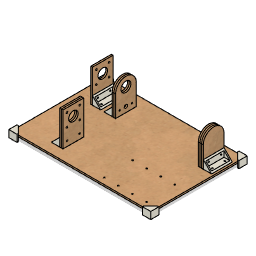
Frame (Autodesk Fusion 360 design; units mm, degrees)
Autodesk Fusion 360 part; units mm, degrees
note: some values were not read from the file. Chosen so that the rebuilt part matches the saved one: a direction; where a step ends. Set by a fixed rule: which sketch regions a step uses.
(part 1 of 2)
sketch "Sketch1" plane through (0, 0, 0) normal (0, 1, 0) x (1, 0, 0)
  line L0 (-148.1327, 87.8458) -> (188.6673, 87.8458)
  line L1 (188.6673, 87.8458) -> (188.6673, -139.1542)
  line L2 (188.6673, -139.1542) -> (-148.1327, -139.1542)
  line L3 (-148.1327, -139.1542) -> (-148.1327, 87.8458)
  line L4 (400.9033, 37.8458) -> (350, 37.8458) construction
  line L5 (350, 37.8458) -> (-250, 37.8458) construction
  line L6 (400, -89.1542) -> (-263.6567, -89.1542) construction
  line L7 (151.7073, 62.8058) -> (163.6273, 62.8058)
  line L8 (163.6273, 62.8058) -> (163.6273, 12.8858)
  line L9 (163.6273, 12.8858) -> (151.7073, 12.8858)
  line L10 (151.7073, 12.8858) -> (151.7073, 62.8058)
  line L11 (-56.2127, 62.8058) -> (-48.2927, 62.8058)
  line L12 (-48.2927, 62.8058) -> (-48.2927, 12.8858)
  line L13 (-48.2927, 12.8858) -> (-56.2127, 12.8858)
  line L14 (-56.2127, 12.8858) -> (-56.2127, 62.8058)
  line L15 (-108.1327, 62.8058) -> (-104.2127, 62.8058)
  line L16 (-104.2127, 62.8058) -> (-104.2127, 12.8858)
  line L17 (-104.2127, 12.8858) -> (-108.1327, 12.8858)
  line L18 (-108.1327, 12.8858) -> (-108.1327, 62.8058)
  line L19 (-56.2127, -64.1942) -> (-48.2927, -64.1942)
  line L20 (-48.2927, -64.1942) -> (-48.2927, -114.1142)
  line L21 (-48.2927, -114.1142) -> (-56.2127, -114.1142)
  line L22 (-56.2127, -114.1142) -> (-56.2127, -64.1942)
  line L23 (155.7073, -64.1942) -> (163.6273, -64.1942)
  line L24 (163.6273, -64.1942) -> (163.6273, -114.1142)
  line L25 (163.6273, -114.1142) -> (155.7073, -114.1142)
  line L26 (155.7073, -114.1142) -> (155.7073, -64.1942)
  line L27 (-108.1327, 46.2192) -> (-104.2127, 46.2192)
  line L28 (-104.2127, 46.2192) -> (-104.2127, 29.4725)
  line L29 (-104.2127, 29.4725) -> (-108.1327, 29.4725)
  line L30 (-108.1327, 29.4725) -> (-108.1327, 46.2192)
  line L31 (-56.2127, 46.2192) -> (-48.2927, 46.2192)
  line L32 (-48.2927, 46.2192) -> (-48.2927, 29.4725)
  line L33 (-48.2927, 29.4725) -> (-56.2127, 29.4725)
  line L34 (-56.2127, 29.4725) -> (-56.2127, 46.2192)
  line L35 (151.7073, 46.2192) -> (163.6273, 46.2192)
  line L36 (163.6273, 46.2192) -> (163.6273, 29.4725)
  line L37 (163.6273, 29.4725) -> (151.7073, 29.4725)
  line L38 (151.7073, 29.4725) -> (151.7073, 46.2192)
  line L39 (-56.2127, -80.7808) -> (-48.2927, -80.7808)
  line L40 (-48.2927, -80.7808) -> (-48.2927, -97.5275)
  line L41 (-48.2927, -97.5275) -> (-56.2127, -97.5275)
  line L42 (-56.2127, -97.5275) -> (-56.2127, -80.7808)
  line L43 (155.7073, -80.7808) -> (163.6273, -80.7808)
  line L44 (163.6273, -80.7808) -> (163.6273, -97.5275)
  line L45 (163.6273, -97.5275) -> (155.7073, -97.5275)
  line L46 (155.7073, -97.5275) -> (155.7073, -80.7808)
  dimension "d4" = 127
  dimension "d5" = 50
  dimension "d6" = 50
  dimension "d7" = 7.92
  dimension "d8" = 11.92
  dimension "d9" = 7.92
  dimension "d10" = 7.92
  dimension "d12" = 49.92
  dimension "d13" = 49.92
  dimension "d14" = 49.92
  dimension "d15" = 49.92
  dimension "d16" = 49.92
  dimension "d17" = 3.92
  dimension "d18" = 24.96
  dimension "d19" = 24.96
  dimension "d20" = 24.96
  dimension "d21" = 24.96
  dimension "d22" = 24.96
  dimension "d23" = 25.04
  dimension "d24" = 7.92
  dimension "d25" = 200
  dimension "d26" = 25.04
  dimension "d27" = 40
  dimension "d28" = 48
  dimension "d455" = 16.7467
  dimension "d456" = 16.5867
  dimension "d457" = 16.7467
  dimension "d458" = 16.5867
  dimension "d459" = 16.7467
  dimension "d460" = 16.5867
  dimension "d461" = 16.5867
  dimension "d462" = 16.7467
  dimension "d463" = 16.5867
  dimension "d464" = 16.7467
  constraint horizontal L0
  constraint vertical L1
  constraint horizontal L2
  constraint vertical L3
  constraint perpendicular L1 L4
  constraint perpendicular L1 L5
  constraint perpendicular L3 L6
  constraint horizontal L7
  constraint vertical L8
  constraint horizontal L9
  constraint vertical L10
  constraint horizontal L11
  constraint vertical L12
  constraint horizontal L13
  constraint vertical L14
  constraint horizontal L15
  constraint vertical L16
  constraint horizontal L17
  constraint vertical L18
  constraint horizontal L19
  constraint vertical L20
  constraint horizontal L21
  constraint vertical L22
  constraint horizontal L23
  constraint vertical L24
  constraint horizontal L25
  constraint vertical L26
  constraint horizontal L27
  constraint vertical L28
  constraint horizontal L29
  constraint vertical L30
  constraint coincident L16 L28.end
  constraint coincident L18 L27.start
  constraint horizontal L31
  constraint vertical L32
  constraint horizontal L33
  constraint vertical L34
  constraint coincident L12 L32.end
  constraint coincident L14 L31.start
  constraint horizontal L35
  constraint vertical L36
  constraint horizontal L37
  constraint vertical L38
  constraint coincident L8 L36.end
  constraint coincident L10 L35.start
  constraint horizontal L39
  constraint vertical L40
  constraint horizontal L41
  constraint vertical L42
  constraint coincident L20 L40.end
  constraint coincident L22 L39.start
  constraint horizontal L43
  constraint vertical L44
  constraint horizontal L45
  constraint vertical L46
  constraint coincident L24 L44.end
  constraint coincident L26 L43.start
  measures "d4" distance of L5 L6
  measures "d5" distance of L2 L6
  measures "d6" distance of L0 L4.end
  measures "d7" distance of L23.start L23.end
  measures "d8" distance of L7.start L7.end
  measures "d9" distance of L11.start L11.end
  measures "d10" distance of L19.start L19.end
  measures "d12" distance of L7.end L8.end
  measures "d13" distance of L23.end L24.end
  measures "d14" distance of L19.end L20.end
  measures "d15" distance of L11.end L12.end
  measures "d16" distance of L15.end L16.end
  measures "d17" distance of L15.start L15.end
  measures "d18" distance of L5 L15.end
  measures "d19" distance of L5 L11.end
  measures "d20" distance of L5 L7.end
  measures "d21" distance of L6 L19.end
  measures "d22" distance of L6 L23.end
  measures "d23" distance of L1 L24
  measures "d24" horizontal distance of L13.end L19.end
  measures "d25" distance of L10 L12
  measures "d26" distance of L1 L8
  measures "d27" distance of L3 L18
  measures "d28" distance of L14 L16
  measures "d455" distance of L27 L29
  measures "d456" distance of L15 L27
  measures "d457" distance of L27 L33
  measures "d458" distance of L11 L31
  measures "d459" distance of L35 L37
  measures "d460" distance of L7.start L35
  measures "d461" distance of L19 L39
  measures "d462" distance of L39 L41
  measures "d463" distance of L23 L43
  measures "d464" distance of L43 L45
extrude "Extrude1" add sketch "Sketch1" along normal blind 4 contours L0 L1 L2 L3 | L8 L10 L35 L36 L37 L38 | L12 L14 L31 L32 L33 L34 | L16 L18 L27 L28 L29 L30 | L20 L22 L39 L40 L41 L42 | L23 L24 L26 L43 | L24 L26 L43 L44 L45 L46 | L24 L25 L26 L45 makes body 1
sketch "Sketch2" plane through (0, 4, 0) normal (0, 1, 0) x (-1, 0, 0)
  line L0 (-163.6273, -12.8858) -> (-151.7073, -12.8858)
  line L1 (-151.7073, -46.2192) -> (-151.7073, -62.8058)
  line L2 (-151.7073, -62.8058) -> (-163.6273, -62.8058)
  line L3 (-163.6273, -62.8058) -> (-163.6273, -46.2192)
  line L4 (48.2927, -12.8858) -> (56.2127, -12.8858)
  line L5 (56.2127, -12.8858) -> (56.2127, -29.4725)
  line L6 (56.2127, -62.8058) -> (48.2927, -62.8058)
  line L7 (48.2927, -29.4725) -> (48.2927, -12.8858)
  line L8 (104.2127, -12.8858) -> (108.1327, -12.8858)
  line L9 (108.1327, -46.2192) -> (108.1327, -62.8058)
  line L10 (108.1327, -62.8058) -> (104.2127, -62.8058)
  line L11 (104.2127, -62.8058) -> (104.2127, -46.2192)
  line L12 (48.2927, 114.1142) -> (56.2127, 114.1142)
  line L13 (56.2127, 114.1142) -> (56.2127, 97.5275)
  line L14 (56.2127, 64.1942) -> (48.2927, 64.1942)
  line L15 (48.2927, 97.5275) -> (48.2927, 114.1142)
  line L16 (148.1327, 139.1542) -> (-188.6673, 139.1542)
  line L17 (-188.6673, 139.1542) -> (-188.6673, -87.8458)
  line L18 (-188.6673, -87.8458) -> (148.1327, -87.8458)
  line L19 (148.1327, -87.8458) -> (148.1327, 139.1542)
  line L20 (-243.4982, -14.4378) -> (-263.4982, -14.4378)
  line L21 (-263.4982, -14.4378) -> (-263.4982, 5.5622)
  line L22 (-263.4982, 5.5622) -> (-243.4982, 5.5622)
  line L23 (-243.4982, 5.5622) -> (-243.4982, -14.4378)
  line L24 (104.2127, -46.2192) -> (108.1327, -46.2192)
  line L25 (104.2127, -29.4725) -> (104.2127, -12.8858)
  line L26 (108.1327, -12.8858) -> (108.1327, -29.4725)
  line L27 (108.1327, -29.4725) -> (104.2127, -29.4725)
  line L28 (56.2127, -29.4725) -> (48.2927, -29.4725)
  line L29 (56.2127, -46.2192) -> (56.2127, -62.8058)
  line L30 (48.2927, -62.8058) -> (48.2927, -46.2192)
  line L31 (48.2927, -46.2192) -> (56.2127, -46.2192)
  line L32 (-163.6273, -46.2192) -> (-151.7073, -46.2192)
  line L33 (-163.6273, -29.4725) -> (-163.6273, -12.8858)
  line L34 (-151.7073, -12.8858) -> (-151.7073, -29.4725)
  line L35 (-151.7073, -29.4725) -> (-163.6273, -29.4725)
  line L36 (56.2127, 97.5275) -> (48.2927, 97.5275)
  line L37 (56.2127, 80.7808) -> (56.2127, 64.1942)
  line L38 (48.2927, 64.1942) -> (48.2927, 80.7808)
  line L39 (48.2927, 80.7808) -> (56.2127, 80.7808)
  dimension "d32" = 20
  dimension "d33" = 20
  constraint horizontal L20
  constraint vertical L21
  constraint horizontal L22
  constraint vertical L23
  measures "d32" distance of L20.start L20.end
  measures "d33" distance of L20.start L22.end
extrude "Extrude2" add sketch "Sketch2" along normal blind 17 separate body contours L20 L21 L22 L23 makes body 2
chamfer "Chamfer1" distance 17 angle 45 1 edges at (263.4982, 12.5, 5.5622) on bodies 2
sketch "Sketch3" plane through (0, 21, 0) normal (0, 1, 0) x (-1, 0, 0)
  line L0 (-246.4982, 5.5622) -> (-263.4982, -11.4378)
  line L1 (-263.4982, -11.4378) -> (-263.4982, -14.4378)
  line L2 (-263.4982, -14.4378) -> (-243.4982, -14.4378)
  line L3 (-243.4982, -14.4378) -> (-243.4982, 5.5622)
  line L4 (-243.4982, 5.5622) -> (-246.4982, 5.5622)
  line L5 (-246.4982, -11.4378) -> (-266.4982, -11.4378)
  line L6 (-266.4982, -11.4378) -> (-266.4982, 8.5622)
  line L7 (-266.4982, 8.5622) -> (-246.4982, 8.5622)
  line L8 (-246.4982, 8.5622) -> (-246.4982, -11.4378)
  dimension "d37" = 3
  dimension "d38" = 3
  dimension "d39" = 20
  dimension "d40" = 20
  constraint horizontal L5
  constraint vertical L6
  constraint horizontal L7
  constraint vertical L8
  measures "d37" distance of L2 L5
  measures "d38" distance of L3 L8
  measures "d39" distance of L6.end L7.end
  measures "d40" distance of L5.end L6.end
extrude "Extrude3" cut sketch "Sketch3" against normal blind 4 from surface at -3 contours L0 L5 L8 | L0 L5 L6 L7 L8 bodies 2
sketch "Sketch4" plane through (0, 4, 0) normal (0, 1, 0) x (-1, 0, 0)
  line L0 (-163.6273, -12.8858) -> (-151.7073, -12.8858)
  line L1 (-151.7073, -46.2192) -> (-151.7073, -62.8058)
  line L2 (-151.7073, -62.8058) -> (-163.6273, -62.8058)
  line L3 (-163.6273, -62.8058) -> (-163.6273, -46.2192)
  line L4 (48.2927, -12.8858) -> (56.2127, -12.8858)
  line L5 (56.2127, -12.8858) -> (56.2127, -29.4725)
  line L6 (56.2127, -62.8058) -> (48.2927, -62.8058)
  line L7 (48.2927, -29.4725) -> (48.2927, -12.8858)
  line L8 (104.2127, -12.8858) -> (108.1327, -12.8858)
  line L9 (108.1327, -46.2192) -> (108.1327, -62.8058)
  line L10 (108.1327, -62.8058) -> (104.2127, -62.8058)
  line L11 (104.2127, -62.8058) -> (104.2127, -46.2192)
  line L12 (48.2927, 114.1142) -> (56.2127, 114.1142)
  line L13 (56.2127, 114.1142) -> (56.2127, 97.5275)
  line L14 (56.2127, 64.1942) -> (48.2927, 64.1942)
  line L15 (48.2927, 97.5275) -> (48.2927, 114.1142)
  line L16 (148.1327, 139.1542) -> (-188.6673, 139.1542)
  line L17 (-188.6673, 139.1542) -> (-188.6673, -87.8458)
  line L18 (-188.6673, -87.8458) -> (148.1327, -87.8458)
  line L19 (148.1327, -87.8458) -> (148.1327, 139.1542)
  line L20 (-250, 50) -> (-270, 50)
  line L21 (-270, 50) -> (-270, 70)
  line L22 (-270, 70) -> (-250, 70)
  line L23 (-250, 70) -> (-250, 50)
  line L24 (104.2127, -46.2192) -> (108.1327, -46.2192)
  line L25 (104.2127, -29.4725) -> (104.2127, -12.8858)
  line L26 (108.1327, -12.8858) -> (108.1327, -29.4725)
  line L27 (108.1327, -29.4725) -> (104.2127, -29.4725)
  line L28 (56.2127, -29.4725) -> (48.2927, -29.4725)
  line L29 (56.2127, -46.2192) -> (56.2127, -62.8058)
  line L30 (48.2927, -62.8058) -> (48.2927, -46.2192)
  line L31 (48.2927, -46.2192) -> (56.2127, -46.2192)
  line L32 (-163.6273, -46.2192) -> (-151.7073, -46.2192)
  line L33 (-163.6273, -29.4725) -> (-163.6273, -12.8858)
  line L34 (-151.7073, -12.8858) -> (-151.7073, -29.4725)
  line L35 (-151.7073, -29.4725) -> (-163.6273, -29.4725)
  line L36 (56.2127, 97.5275) -> (48.2927, 97.5275)
  line L37 (56.2127, 80.7808) -> (56.2127, 64.1942)
  line L38 (48.2927, 64.1942) -> (48.2927, 80.7808)
  line L39 (48.2927, 80.7808) -> (56.2127, 80.7808)
  dimension "d44" = 20
  dimension "d45" = 20
  constraint horizontal L20
  constraint vertical L21
  constraint horizontal L22
  constraint vertical L23
  measures "d44" distance of L20.start L20.end
  measures "d45" distance of L20.start L22.end
extrude "Extrude4" add sketch "Sketch4" along normal blind 10 separate body contours L20 L21 L22 L23 makes body 3
sketch "Sketch5" plane through (0, 14, 0) normal (0, 1, 0) x (-1, 0, 0)
  line L0 (-250, 70) -> (-270, 70)
  line L1 (-270, 70) -> (-270, 50)
  line L2 (-270, 50) -> (-250, 50)
  line L3 (-250, 50) -> (-250, 70)
  circle A0 centre (-260, 60) radius 1.75
  line L4 (-250, 50) -> (-270, 70) construction
  dimension "d48" = 3.5
  constraint coincident L2.end L3.start
  constraint coincident L0.end L1.start
  constraint midpoint A0.centre L4
  measures "d48" diameter of A0
sketch "Sketch6" plane through (270, 0, 0) normal (1, 0, 0) x (0, 0, -1)
  line L0 (-70, 4) -> (-50, 4)
  line L1 (-50, 4) -> (-50, 14)
  line L2 (-50, 14) -> (-70, 14)
  line L3 (-70, 14) -> (-70, 4)
  line L4 (-62.9, 11) -> (-57.1, 11)
  line L5 (-57.1, 11) -> (-57.1, 7.6)
  line L6 (-57.1, 7.6) -> (-62.9, 7.6)
  line L7 (-62.9, 7.6) -> (-62.9, 11)
  line L8 (-60, 14) -> (-60, 4) construction
  line L9 (-50, 14) -> (-70, 14) construction
  dimension "d49" = 5.8
  dimension "d50" = 3.4
  dimension "d51" = 7.1
  dimension "d52" = 3
  constraint horizontal L4
  constraint vertical L5
  constraint horizontal L6
  constraint vertical L7
  constraint midpoint L2 L8.start
  constraint midpoint L0 L8.end
  measures "d49" distance of L4.start L4.end
  measures "d50" distance of L4.end L5.end
  measures "d51" distance of L3 L7
  measures "d52" distance of L4 L9
extrude "Extrude5" cut sketch "Sketch6" against normal blind 13.3 contours L4 L5 L6 L7 bodies 3
extrude "Extrude6" cut sketch "Sketch5" against normal up to surface (6.4 mm away) contours A0 bodies 3
sketch "Sketch7" plane through (0, 0, 0) normal (1, 0, 0) x (0, 0, -1)
  line L0 (179.5513, 0) -> (229.4713, 0)
  line L1 (229.4713, 0) -> (229.4713, 83.5)
  line L2 (229.4713, 83.5) -> (179.5513, 83.5)
  line L3 (179.5513, 83.5) -> (179.5513, 0)
  line L4 (179.5513, 58) -> (229.4713, 58) construction
  circle A0 centre (204.5113, 58) radius 11.46
  circle A1 centre (189.0113, 73.5) radius 1.96
  circle A2 centre (220.0113, 73.5) radius 1.96
  circle A3 centre (220.0113, 42.5) radius 1.96
  circle A4 centre (189.0113, 42.5) radius 1.96
  line L5 (189.0113, 73.5) -> (220.0113, 42.5) construction
  line L6 (179.5513, 4) -> (229.4713, 4) construction
  dimension "d58" = 22.92
  dimension "d59" = 3.92
  dimension "d60" = 3.92
  dimension "d61" = 3.92
  dimension "d62" = 3.92
  dimension "d63" = 31
  dimension "d64" = 31
  dimension "d65" = 31
  dimension "d66" = 31
  dimension "d67" = 31
  dimension "d68" = 31
  dimension "d69" = 49.92
  dimension "d70" = 15.5
  dimension "d71" = 4
  dimension "d72" = 54
  dimension "d73" = 10
  dimension "d74" = 15.5
  dimension "d125" = 58
  constraint horizontal L0
  constraint vertical L1
  constraint horizontal L2
  constraint vertical L3
  constraint coincident L3 L4.start
  constraint coincident L1 L4.end
  constraint perpendicular L1 L4
  constraint midpoint L4 A0.centre
  constraint coincident A1.centre L5.start
  constraint coincident A3.centre L5.end
  constraint coincident L3 L6.start
  constraint coincident L1 L6.end
  constraint perpendicular L1 L6
  measures "d58" diameter of A0
  measures "d59" diameter of A4
  measures "d60" diameter of A1
  measures "d61" diameter of A2
  measures "d62" diameter of A3
  measures "d63" distance of A1.centre A2.centre
  measures "d64" horizontal distance of A3.centre A4.centre
  measures "d65" vertical distance of A2.centre A3.centre
  measures "d66" vertical distance of A1.centre A4.centre
  measures "d67" horizontal distance of A2.centre A4.centre
  measures "d68" vertical distance of A1.centre A3.centre
  measures "d69" distance of L1.end L2.end
  measures "d70" horizontal distance of A0.centre A2.centre
  measures "d71" distance of L0 L6
  measures "d72" distance of A0.centre L6
  measures "d73" distance of L2 A2.centre
  measures "d74" vertical distance of A0.centre A2.centre
  measures "d125" vertical distance of origin A0.centre
extrude "Extrude7" add sketch "Sketch7" along normal blind 4 separate body makes body 4
sketch "Sketch8" plane through (0, 0, 0) normal (1, 0, 0) x (0, 0, -1)
  line L0 (256.2856, 0) -> (306.2056, 0)
  line L1 (306.2056, 0) -> (306.2056, 55.0081)
  line L2 (256.2856, 55.0081) -> (256.2856, 0)
  line L3 (256.2856, 4) -> (306.2056, 4) construction
  circle A0 centre (281.2456, 58) radius 11.96
  arc A1 (281.883, 79.96) -> (256.2856, 55.0081) centre (281.2456, 55.0081) ccw
  arc A2 (306.2056, 55.0081) -> (281.883, 79.96) centre (281.2456, 55.0081) ccw
  line L4 (256.2856, 77.8525) -> (306.2056, 77.8525) construction
  circle A3 centre (281.2456, 17) radius 4
  point P0 (306.2056, 77.8525)
  point P1 (256.2856, 77.8525)
  dimension "d77" = 4
  dimension "d78" = 49.92
  dimension "d80" = 23.92
  dimension "d81" = 54
  dimension "d83" = 24.96
  dimension "d84" = 24.96
  dimension "d85" = 49.92
  dimension "d86" = 49.92
  dimension "d87" = 21.96
  dimension "d88" = 24.96
  dimension "d124" = 58
  dimension "d520" = 24.96
  dimension "d521" = 8
  dimension "d522" = 13
  constraint horizontal L0
  constraint vertical L1
  constraint vertical L2
  constraint coincident L2 L3.start
  constraint coincident L1 L3.end
  constraint perpendicular L1 L3
  constraint coincident P1 L2
  constraint tangent L2 A1
  constraint coincident P0 L1
  constraint tangent L1 A2
  constraint coincident A1.start A2.end
  constraint coincident P1 L4.start
  constraint coincident P0 L4.end
  constraint perpendicular L1 L4
  measures "d77" distance of L0 L3
  measures "d78" distance of P0 P1
  measures "d80" diameter of A0
  measures "d81" distance of L3 A0.centre
  measures "d83" radius of A1
  measures "d84" radius of A2
  measures "d85" distance of P1 L1
  measures "d86" horizontal distance of P0 L2.start
  measures "d87" vertical distance of A0.centre A1.start
  measures "d88" distance of L1 A0.centre
  measures "d124" vertical distance of origin A0.centre
  measures "d520" distance of L1 A3.centre
  measures "d521" diameter of A3
  measures "d522" distance of L3 A3.centre
extrude "Extrude8" add sketch "Sketch8" along normal blind 4 separate body makes body 5
extrude "Extrude22" add sketch "Sketch8" 1 faces at (0, 24.3957, -263.3315) along normal blind 4 separate body contours A0 | A3 on bodies 5 makes body 6
move_body "Move1" bodies 6 to x (1, 0, 0) y (0, 1, 0) z (0, 0, 1) at (0, 0, -70)
extrude "Extrude24" add sketch "Sketch8" along normal blind 4 separate body contours L0 L1 L2 A1 A2 | A3 makes body 7
move_body "Move2" bodies 7 to x (1, 0, 0) y (0, 1, 0) z (0, 0, 1) at (0, 0, -135)
sketch "Sketch9" plane through (0, 0, 0) normal (1, 0, 0) x (0, 0, -1)
  line L0 (-160, 0) -> (-209.92, 0)
  line L1 (-209.92, 0) -> (-209.92, 51)
  line L2 (-160, 51) -> (-160, 0)
  line L3 (-209.92, 4) -> (-160, 4) construction
  circle A0 centre (-184.96, 60) radius 5.96
  arc A1 (-184.96, 75.96) -> (-209.92, 51) centre (-184.96, 51) ccw
  arc A2 (-160, 51) -> (-184.96, 75.96) centre (-184.96, 51) ccw
  dimension "d91" = 4
  dimension "d92" = 49.92
  dimension "d94" = 11.92
  dimension "d95" = 56
  dimension "d98" = 24.96
  dimension "d99" = 24.96
  dimension "d100" = 15.96
  dimension "d101" = 24.96
  constraint horizontal L0
  constraint vertical L1
  constraint vertical L2
  constraint coincident L1 L3.start
  constraint coincident L2 L3.end
  constraint perpendicular L2 L3
  constraint tangent L1 A1
  constraint tangent L2 A2
  constraint coincident A1.start A2.end
  measures "d91" distance of L0 L3
  measures "d92" distance of L0.start L0.end
  measures "d94" diameter of A0
  measures "d95" distance of L3 A0.centre
  measures "d98" radius of A1
  measures "d99" radius of A2
  measures "d100" distance of A0.centre A1.start
  measures "d101" distance of L2 A0.centre
extrude "Extrude9" add sketch "Sketch9" along normal blind 4 separate body makes body 8
sketch "Sketch10" plane through (0, 0, 0) normal (1, 0, 0) x (0, 0, -1)
  line L0 (-240, 0) -> (-289.92, 0)
  line L1 (-289.92, 0) -> (-289.92, 85.5)
  line L2 (-289.92, 85.5) -> (-240, 85.5)
  line L3 (-240, 85.5) -> (-240, 0)
  line L4 (-289.92, 4) -> (-240, 4) construction
  circle A0 centre (-264.96, 60) radius 11.46
  circle A1 centre (-249.46, 75.5) radius 1.96
  circle A2 centre (-249.46, 44.5) radius 1.96
  circle A3 centre (-280.46, 44.5) radius 1.96
  circle A4 centre (-280.46, 75.5) radius 1.96
  dimension "d104" = 4
  dimension "d105" = 22.92
  dimension "d106" = 3.92
  dimension "d107" = 31
  dimension "d108" = 3.92
  dimension "d109" = 3.92
  dimension "d110" = 3.92
  dimension "d111" = 31
  dimension "d112" = 31
  dimension "d113" = 31
  dimension "d114" = 31
  dimension "d115" = 31
  dimension "d116" = 15.5
  dimension "d117" = 15.5
  dimension "d118" = 56
  dimension "d119" = 10
  dimension "d120" = 49.92
  dimension "d121" = 24.96
  constraint horizontal L0
  constraint vertical L1
  constraint horizontal L2
  constraint vertical L3
  constraint coincident L1 L4.start
  constraint coincident L3 L4.end
  constraint perpendicular L3 L4
  measures "d104" distance of L0 L4
  measures "d105" diameter of A0
  measures "d106" diameter of A1
  measures "d107" vertical distance of A1.centre A2.centre
  measures "d108" diameter of A3
  measures "d109" diameter of A2
  measures "d110" diameter of A4
  measures "d111" horizontal distance of A1.centre A4.centre
  measures "d112" horizontal distance of A2.centre A3.centre
  measures "d113" vertical distance of A3.centre A4.centre
  measures "d114" vertical distance of A1.centre A3.centre
  measures "d115" horizontal distance of A2.centre A4.centre
  measures "d116" horizontal distance of A0.centre A1.centre
  measures "d117" vertical distance of A0.centre A3.centre
  measures "d118" distance of L4 A0.centre
  measures "d119" distance of L2 A1.centre
  measures "d120" distance of L0.start L0.end
  measures "d121" distance of L3 A0.centre
extrude "Extrude10" add sketch "Sketch10" along normal blind 4 separate body makes body 9
sketch "Sketch11" plane through (0, 0, 0) normal (0, 0, 1) x (1, 0, 0)
  line L0 (295.5184, 4) -> (315.5184, 4)
  line L1 (315.5184, 4) -> (295.5184, 24)
  line L2 (295.5184, 24) -> (295.5184, 4)
  line L3 (298.5184, 21) -> (298.5184, 7)
  line L4 (298.5184, 7) -> (312.5184, 7)
  dimension "d126" = 45
  dimension "d127" = 20
  dimension "d128" = 4
  dimension "d129" = 3
  dimension "d130" = 3
  constraint horizontal L0
  constraint perpendicular L0 L2
  constraint coincident L1 L3.start
  constraint vertical L3
  constraint coincident L1 L4.end
  constraint perpendicular L3 L4
  measures "d126" angle of L0 L1
  measures "d127" distance of L0.start L0.end
  measures "d128" distance of origin L0
  measures "d129" distance of L0 L4
  measures "d130" distance of L2 L3
extrude "Extrude11" add sketch "Sketch11" along normal blind 3 separate body makes body 10
extrude "Extrude12" add sketch "Sketch11" along normal blind 50 contours L0 L1 L2 L3 L4 bodies 10
extrude "Extrude13" add sketch "Sketch11" against normal blind 3 from surface at 50 bodies 10
sketch "Sketch12" plane through (298.5184, 0, 0) normal (1, 0, 0) x (0, 0, -1)
  line L0 (-47, 21) -> (-47, 7)
  line L1 (-47, 7) -> (-3, 7)
  line L2 (-3, 7) -> (-3, 21)
  line L3 (-3, 21) -> (-47, 21)
  circle A0 centre (-10, 16) radius 1.75
  circle A1 centre (-40, 16) radius 1.75
  line L4 (-25, 21) -> (-25, 7) construction
  line L5 (-50, 4) -> (-50, 24)
  point P0 (-50, 4)
  dimension "d138" = 3.5
  dimension "d139" = 3.5
  dimension "d149" = 12
  dimension "d150" = 30
  dimension "d151" = 15
  dimension "d152" = 12
  constraint midpoint L3 L4.start
  constraint midpoint L1 L4.end
  measures "d138" diameter of A1
  measures "d139" diameter of A0
  measures "d149" vertical distance of A1.centre P0
  measures "d150" distance of A0.centre A1.centre
  measures "d151" distance of A1.centre L4
  measures "d152" vertical distance of A0.centre P0
extrude "Extrude14" cut sketch "Sketch12" against normal up to surface (3 mm away) contours A0 | A1 bodies 10
sketch "Sketch13" plane through (0, 7, 0) normal (0, 1, 0) x (-1, 0, 0)
  line L0 (-298.5184, 47) -> (-312.5184, 47)
  line L1 (-312.5184, 47) -> (-312.5184, 3)
  line L2 (-312.5184, 3) -> (-298.5184, 3)
  line L3 (-298.5184, 3) -> (-298.5184, 47)
  circle A0 centre (-307.5184, 10) radius 1.75
  circle A1 centre (-307.5184, 40) radius 1.75
  line L4 (-315.5184, 0) -> (-295.5184, 0)
  line L5 (-315.5184, 0) -> (-315.5184, 50)
  point P0 (-295.5184, 0)
  dimension "d143" = 3.5
  dimension "d144" = 3.5
  dimension "d153" = 10
  dimension "d154" = 30
  dimension "d155" = 50
  dimension "d156" = 12
  dimension "d157" = 12
  measures "d143" diameter of A1
  measures "d144" diameter of A0
  measures "d153" distance of A0.centre L4
  measures "d154" distance of A0.centre A1.centre
  measures "d155" distance of L4.start L5.end
  measures "d156" horizontal distance of A0.centre P0
  measures "d157" horizontal distance of A1.centre P0
extrude "Extrude15" cut sketch "Sketch13" against normal up to surface (3 mm away) contours A0 | A1 bodies 10
sketch "Sketch14" plane through (4, 0, 0) normal (1, 0, 0) x (0, 0, -1)
  circle A0 centre (-249.46, 44.5) radius 1.96
  circle A1 centre (-280.46, 44.5) radius 1.96
  circle A2 centre (-280.46, 75.5) radius 1.96
  circle A3 centre (-249.46, 75.5) radius 1.96
  circle A4 centre (-264.96, 60) radius 11.46
  line L0 (-240, 85.5) -> (-289.92, 85.5)
  line L1 (-289.92, 85.5) -> (-289.92, 0)
  line L2 (-289.92, 0) -> (-240, 0)
  line L3 (-240, 0) -> (-240, 85.5)
  circle A5 centre (-279.96, 16) radius 1.71
  circle A6 centre (-249.96, 16) radius 1.71
  line L4 (-273.2533, 0) -> (-256.6667, 0)
  line L5 (-256.6667, 0) -> (-256.6667, 3.96)
  line L6 (-256.6667, 3.96) -> (-273.2533, 3.96)
  line L7 (-273.2533, 3.96) -> (-273.2533, 0)
  dimension "d160" = 16
  dimension "d161" = 16
  dimension "d162" = 30
  dimension "d163" = 3.42
  dimension "d164" = 3.42
  dimension "d165" = 9.96
  dimension "d166" = 49.92
  dimension "d465" = 3.96
  dimension "d466" = 16.5867
  dimension "d467" = 16.6667
  constraint horizontal L4
  constraint vertical L5
  constraint horizontal L6
  constraint vertical L7
  constraint coincident L2 L4.start
  measures "d160" vertical distance of L1.end A5.centre
  measures "d161" vertical distance of L1.end A6.centre
  measures "d162" distance of A5.centre A6.centre
  measures "d163" diameter of A5
  measures "d164" diameter of A6
  measures "d165" horizontal distance of L1.end A5.centre
  measures "d166" distance of L1.end L2.end
  measures "d465" distance of L4.end L5.end
  measures "d466" distance of L5.end L6.end
  measures "d467" distance of L1.end L4.start
sketch "Sketch15" plane through (4, 0, 0) normal (1, 0, 0) x (0, 0, -1)
  circle A0 centre (-184.96, 60) radius 5.96
  line L0 (-160, 0) -> (-160, 51)
  arc A1 (-160, 51) -> (-209.92, 51) centre (-184.96, 51) ccw
  line L1 (-209.92, 51) -> (-209.92, 0)
  line L2 (-209.92, 0) -> (-160, 0)
  circle A2 centre (-169.875, 16) radius 1.71
  circle A3 centre (-199.875, 16) radius 1.71
  line L3 (-209.75, 0) -> (-160, 0)
  line L4 (-193.1683, 0) -> (-176.5817, 0)
  line L5 (-176.5817, 0) -> (-176.5817, 3.96)
  line L6 (-176.5817, 3.96) -> (-193.1683, 3.96)
  line L7 (-193.1683, 3.96) -> (-193.1683, 0)
  dimension "d167" = 16
  dimension "d168" = 16
  dimension "d169" = 30
  dimension "d170" = 3.42
  dimension "d171" = 3.42
  dimension "d172" = 9.875
  dimension "d174" = 49.75
  dimension "d175" = 49.75
  dimension "d176" = 16
  dimension "d468" = 3.96
  dimension "d469" = 16.5817
  dimension "d470" = 16.5867
  constraint perpendicular L1 L3
  constraint horizontal L4
  constraint vertical L5
  constraint horizontal L6
  constraint vertical L7
  constraint coincident L3 L4.start
  measures "d167" vertical distance of L3.start A3.centre
  measures "d168" vertical distance of L3.start A2.centre
  measures "d169" distance of A3.centre A2.centre
  measures "d170" diameter of A3
  measures "d171" diameter of A2
  measures "d172" horizontal distance of L3.start A3.centre
  measures "d174" distance of L0.start L3.start
  measures "d175" horizontal distance of L0.start L3.start
  measures "d176" vertical distance of L1.end A3.centre
  measures "d468" distance of L4.end L5.end
  measures "d469" distance of L3.start L7
  measures "d470" distance of L4.start L4.end
sketch "Sketch16" plane through (4, 0, 0) normal (1, 0, 0) x (0, 0, -1)
  circle A0 centre (189.0113, 73.5) radius 1.96
  circle A1 centre (204.5113, 58) radius 11.46
  circle A2 centre (220.0113, 73.5) radius 1.96
  circle A3 centre (220.0113, 42.5) radius 1.96
  circle A4 centre (189.0113, 42.5) radius 1.96
  line L0 (179.5513, 83.5) -> (179.5513, 0)
  line L1 (179.5513, 0) -> (229.4713, 0)
  line L2 (229.4713, 0) -> (229.4713, 83.5)
  line L3 (229.4713, 83.5) -> (179.5513, 83.5)
  circle A5 centre (219.5113, 16) radius 1.71
  circle A6 centre (189.5113, 16) radius 1.71
  line L4 (196.2179, 0) -> (212.8046, 0)
  line L5 (212.8046, 0) -> (212.8046, 3.96)
  line L6 (212.8046, 3.96) -> (196.2179, 3.96)
  line L7 (196.2179, 3.96) -> (196.2179, 0)
  dimension "d179" = 30
  dimension "d180" = 3.42
  dimension "d181" = 3.42
  dimension "d185" = 16
  dimension "d364" = 49.92
  dimension "d365" = 9.96
  dimension "d366" = 16
  dimension "d471" = 3.96
  dimension "d472" = 16.6667
  dimension "d473" = 16.5867
  constraint horizontal L4
  constraint vertical L5
  constraint horizontal L6
  constraint vertical L7
  constraint coincident L1 L4.start
  measures "d179" distance of A6.centre A5.centre
  measures "d180" diameter of A6
  measures "d181" diameter of A5
  measures "d185" vertical distance of L0.end A6.centre
  measures "d364" distance of L0.end L1.end
  measures "d365" horizontal distance of L0.end A6.centre
  measures "d366" vertical distance of L1.end A5.centre
  measures "d471" distance of L4 L6
  measures "d472" distance of L0.end L4.start
  measures "d473" distance of L5.end L6.end
sketch "Sketch17" plane through (4, 0, 0) normal (1, 0, 0) x (0, 0, -1)
  circle A0 centre (281.2456, 58) radius 11.96
  arc A1 (306.2056, 55.0081) -> (256.2856, 55.0081) centre (281.2456, 55.0081) ccw
  line L0 (256.2856, 55.0081) -> (256.2856, 0)
  line L1 (256.2856, 0) -> (306.2056, 0)
  line L2 (306.2056, 0) -> (306.2056, 55.0081)
  circle A2 centre (296.2456, 16) radius 1.71
  circle A3 centre (266.2456, 16) radius 1.71
  line L3 (272.9523, 0) -> (289.5389, 0)
  line L4 (289.5389, 0) -> (289.5389, 3.96)
  line L5 (289.5389, 3.96) -> (272.9523, 3.96)
  line L6 (272.9523, 3.96) -> (272.9523, 0)
  circle A4 centre (281.2456, 17) radius 4
  dimension "d189" = 30
  dimension "d190" = 3.42
  dimension "d191" = 3.42
  dimension "d195" = 16
  dimension "d367" = 49.92
  dimension "d368" = 9.96
  dimension "d369" = 16
  dimension "d474" = 16.5867
  dimension "d475" = 3.96
  dimension "d476" = 16.6667
  constraint horizontal L3
  constraint vertical L4
  constraint horizontal L5
  constraint vertical L6
  constraint coincident L1 L3.start
  measures "d189" distance of A3.centre A2.centre
  measures "d190" diameter of A3
  measures "d191" diameter of A2
  measures "d195" vertical distance of L0.end A3.centre
  measures "d367" distance of L0.end L1.end
  measures "d368" horizontal distance of L0.end A3.centre
  measures "d369" vertical distance of L1.end A2.centre
  measures "d474" distance of L4.end L5.end
  measures "d475" distance of L3 L5
  measures "d476" distance of L0.end L3.start
sketch "Sketch23" plane through (4, 0, 0) normal (1, 0, 0) x (0, 0, -1)
  arc A0 (376.2056, 55.0081) -> (326.2856, 55.0081) centre (351.2456, 55.0081) ccw
  line L0 (326.2856, 55.0081) -> (326.2856, 0)
  line L1 (326.2856, 0) -> (376.2056, 0)
  line L2 (376.2056, 0) -> (376.2056, 55.0081)
  circle A1 centre (336.2456, 16) radius 1.71
  circle A2 centre (366.2456, 16) radius 1.71
  line L3 (342.9523, 0) -> (359.5389, 0)
  line L4 (359.5389, 0) -> (359.5389, 3.96)
  line L5 (359.5389, 3.96) -> (342.9523, 3.96)
  line L6 (342.9523, 3.96) -> (342.9523, 0)
  dimension "d323" = 3.42
  dimension "d324" = 3.42
  dimension "d325" = 30
  dimension "d326" = 16
  dimension "d327" = 16
  dimension "d328" = 9.96
  dimension "d329" = 49.92
  dimension "d477" = 3.96
  dimension "d478" = 16.6667
  dimension "d479" = 16.5867
  constraint horizontal L3
  constraint vertical L4
  constraint horizontal L5
  constraint vertical L6
  constraint coincident L1 L3.start
  measures "d323" diameter of A2
  measures "d324" diameter of A1
  measures "d325" horizontal distance of A1.centre A2.centre
  measures "d326" vertical distance of L1.end A2.centre
  measures "d327" vertical distance of L0.end A1.centre
  measures "d328" horizontal distance of L0.end A1.centre
  measures "d329" distance of L0.end L1.end
  measures "d477" distance of L3 L5
  measures "d478" distance of L0 L6
  measures "d479" distance of L4.end L5.end
sketch "Sketch24" plane through (4, 0, 0) normal (1, 0, 0) x (0, 0, -1)
  circle A0 centre (416.2456, 58) radius 11.96
  arc A1 (441.2056, 55.0081) -> (391.2856, 55.0081) centre (416.2456, 55.0081) ccw
  line L0 (391.2856, 55.0081) -> (391.2856, 0)
  line L1 (391.2856, 0) -> (441.2056, 0)
  line L2 (441.2056, 0) -> (441.2056, 55.0081)
  circle A2 centre (401.2456, 16) radius 1.71
  circle A3 centre (431.2456, 16) radius 1.71
  line L3 (407.9523, 0) -> (424.5389, 0)
  line L4 (424.5389, 0) -> (424.5389, 3.96)
  line L5 (424.5389, 3.96) -> (407.9523, 3.96)
  line L6 (407.9523, 3.96) -> (407.9523, 0)
  dimension "d525" = 16
  dimension "d526" = 16
  dimension "d527" = 3.42
  dimension "d528" = 3.42
  dimension "d529" = 30
  dimension "d530" = 49.92
  dimension "d531" = 9.96
  dimension "d532" = 16.5867
  dimension "d533" = 3.96
  dimension "d534" = 16.6667
  constraint horizontal L3
  constraint vertical L4
  constraint horizontal L5
  constraint vertical L6
  constraint coincident L1 L3.start
  measures "d525" distance of L1 A2.centre
  measures "d526" distance of L1 A3.centre
  measures "d527" diameter of A2
  measures "d528" diameter of A3
  measures "d529" distance of A2.centre A3.centre
  measures "d530" distance of L0.end L1.end
  measures "d531" horizontal distance of L0.end A2.centre
  measures "d532" distance of L4.end L5.end
  measures "d533" distance of L3 L5
  measures "d534" distance of L0.end L3.start
extrude "Extrude16" cut sketch "Sketch15" sketch "Sketch14" sketch "Sketch16" sketch "Sketch17" along normal up to surface contours L2 L3 L4 L5 L6 L7 | A2 | A3 of sketch 2 contours L2 L4 L5 L6 L7 | A5 | A6 of sketch 3 contours L1 L4 L5 L6 L7 | A5 | A6 of sketch 4 contours L1 L3 L4 L5 L6 | A2 | A3 end surface through (0, 0, 0) normal (1, 0, 0) offset 0 bodies 4 5 8 9
extrude "Extrude23" cut sketch "Sketch23" against normal up to surface (4 mm away) contours L1 L3 L4 L5 L6 | A1 | A2 bodies 6
extrude "Extrude25" cut sketch "Sketch24" along normal up to far side of body 7 contours L1 L3 L4 L5 L6 | A2 | A3 bodies 7
sketch "Sketch18" plane through (0, 4, 0) normal (0, 1, 0) x (-1, 0, 0)
  circle A0 centre (92.2127, -52.8458) radius 1.71
  circle A1 centre (92.2127, -22.8458) radius 1.71
  circle A2 centre (68.2127, -22.8458) radius 1.71
  circle A3 centre (68.2127, -52.8458) radius 1.71
  line L0 (104.2127, -29.4725) -> (104.2127, -12.8858) construction
  line L1 (104.2127, -46.2192) -> (104.2127, -29.4725) construction
  line L2 (104.2127, -37.8458) -> (-183.6627, -37.8458) construction
  circle A4 centre (68.2127, 74.1542) radius 1.71
  circle A5 centre (68.2127, 104.1542) radius 1.71
  circle A6 centre (-175.6273, -52.8458) radius 1.71
  circle A7 centre (-175.6273, -22.8458) radius 1.71
  line L3 (-163.6273, -29.4725) -> (-163.6273, -12.8858)
  line L4 (56.2127, 80.7808) -> (56.2127, 97.5275) construction
  line L5 (56.2127, 89.1542) -> (116.1701, 89.1542) construction
  point P0 (108.1327, -46.2192)
  point P1 (108.1327, -29.4725)
  point P2 (-151.7073, -46.2192)
  point P3 (-151.7073, -29.4725)
  point P4 (-163.6273, -29.4725)
  point P5 (-163.6273, -46.2192)
  point P6 (56.2127, -29.4725)
  point P7 (56.2127, -46.2192)
  point P8 (104.2127, -46.2192)
  point P9 (48.2927, 80.7808)
  point P10 (48.2927, 97.5275)
  point P11 (56.2127, 80.7808)
  point P12 (56.2127, 97.5275)
  dimension "d492" = 3.42
  dimension "d493" = 3.42
  dimension "d494" = 3.42
  dimension "d495" = 3.42
  dimension "d496" = 3.42
  dimension "d497" = 3.42
  dimension "d498" = 3.42
  dimension "d499" = 3.42
  dimension "d500" = 12
  dimension "d501" = 12
  dimension "d502" = 12
  dimension "d503" = 12
  dimension "d504" = 12
  dimension "d505" = 12
  dimension "d506" = 12
  dimension "d507" = 12
  dimension "d508" = 15
  dimension "d509" = 15
  dimension "d510" = 15
  dimension "d511" = 15
  dimension "d512" = 15
  dimension "d513" = 15
  dimension "d514" = 15
  dimension "d515" = 15
  constraint coincident P8 L1.start
  constraint coincident L0.start L1.end
  constraint midpoint L1 L2.start
  constraint perpendicular L1 L2
  constraint coincident P11 L4.start
  constraint coincident P12 L4.end
  constraint midpoint L4 L5.start
  constraint perpendicular L4 L5
  measures "d492" diameter of A0
  measures "d493" diameter of A1
  measures "d494" diameter of A3
  measures "d495" diameter of A2
  measures "d496" diameter of A5
  measures "d497" diameter of A4
  measures "d498" diameter of A6
  measures "d499" diameter of A7
  measures "d500" horizontal distance of P5 A6.centre
  measures "d501" distance of A7.centre L3
  measures "d502" horizontal distance of A3.centre P7
  measures "d503" horizontal distance of A0.centre P8
  measures "d504" horizontal distance of A2.centre P6
  measures "d505" horizontal distance of A1.centre L0.start
  measures "d506" horizontal distance of A4.centre P11
  measures "d507" horizontal distance of A5.centre P12
  measures "d508" distance of A4.centre L5
  measures "d509" distance of A5.centre L5
  measures "d510" distance of A1.centre L2
  measures "d511" distance of A0.centre L2
  measures "d512" distance of A3.centre L2
  measures "d513" distance of A2.centre L2
  measures "d514" distance of L2 A6.centre
  measures "d515" distance of L2 A7.centre
extrude "Extrude17" cut sketch "Sketch18" against normal through all bodies 1
sketch "Sketch22" plane through (0, 4, 0) normal (0, 1, 0) x (-1, 0, 0)
  line L0 (48.2927, 114.1142) -> (56.2127, 114.1142)
  line L1 (56.2127, 114.1142) -> (56.2127, 97.5275)
  line L2 (56.2127, 64.1942) -> (48.2927, 64.1942)
  line L3 (48.2927, 97.5275) -> (48.2927, 114.1142)
  line L4 (104.2127, -12.8858) -> (108.1327, -12.8858)
  line L5 (108.1327, -46.2192) -> (108.1327, -62.8058)
  line L6 (108.1327, -62.8058) -> (104.2127, -62.8058)
  line L7 (104.2127, -62.8058) -> (104.2127, -46.2192)
  line L8 (48.2927, -12.8858) -> (56.2127, -12.8858)
  line L9 (56.2127, -12.8858) -> (56.2127, -29.4725)
  line L10 (48.2927, -29.4725) -> (48.2927, -12.8858)
  line L11 (-163.6273, -12.8858) -> (-151.7073, -12.8858)
  line L12 (148.1327, 139.1542) -> (-188.6673, 139.1542)
  line L13 (-188.6673, 139.1542) -> (-188.6673, -87.8458)
  line L14 (-188.6673, -87.8458) -> (148.1327, -87.8458)
  line L15 (148.1327, -87.8458) -> (148.1327, 139.1542)
  circle A0 centre (-59.6994, 53.9542) radius 1.71
  circle A1 centre (-93.6994, 53.9542) radius 1.71
  circle A2 centre (-127.6994, 53.9542) radius 1.71
  circle A3 centre (-161.6994, 53.9542) radius 1.71
  circle A4 centre (-61.5402, 124.3542) radius 1.625
  circle A5 centre (-95.598, 124.3542) radius 1.625
  circle A6 centre (-129.6263, 124.3542) radius 1.625
  circle A7 centre (-163.643, 124.3542) radius 1.625
  line L16 (104.2127, -46.2192) -> (108.1327, -46.2192)
  line L17 (104.2127, -29.4725) -> (104.2127, -12.8858)
  line L18 (108.1327, -12.8858) -> (108.1327, -29.4725)
  line L19 (108.1327, -29.4725) -> (104.2127, -29.4725)
  line L20 (-163.6273, -29.4725) -> (-163.6273, -12.8858)
  line L21 (-151.7073, -12.8858) -> (-151.7073, -29.4725)
  line L22 (56.2127, 97.5275) -> (48.2927, 97.5275)
  line L23 (56.2127, 80.7808) -> (56.2127, 64.1942)
  line L24 (48.2927, 64.1942) -> (48.2927, 80.7808)
  line L25 (48.2927, 80.7808) -> (56.2127, 80.7808)
  line L26 (48.2927, 80.7808) -> (48.2927, 97.5275) construction
  line L27 (48.2927, 89.1542) -> (-188.6673, 89.1542) construction
  circle A8 centre (68.2127, 74.1542) radius 1.71
  circle A9 centre (92.2127, -22.8458) radius 1.71
  circle A10 centre (68.2127, 104.1542) radius 1.71
  circle A11 centre (92.2127, -52.8458) radius 1.71
  dimension "d286" = 3.42
  dimension "d287" = 3.42
  dimension "d288" = 3.42
  dimension "d289" = 3.42
  dimension "d290" = 34
  dimension "d291" = 34
  dimension "d292" = 34
  dimension "d480" = 35.2
  dimension "d481" = 35.2
  dimension "d482" = 35.2
  dimension "d483" = 35.2
  dimension "d484" = 35.2
  dimension "d485" = 35.2
  dimension "d486" = 35.2
  dimension "d487" = 35.2
  constraint coincident L24.end L25.start
  constraint midpoint L26 L27.start
  constraint coincident L13 L27.end
  constraint perpendicular L13 L27
  measures "d286" diameter of A3
  measures "d287" diameter of A2
  measures "d288" diameter of A1
  measures "d289" diameter of A0
  measures "d290" distance of A0.centre A1.centre
  measures "d291" horizontal distance of A1.centre A2.centre
  measures "d292" horizontal distance of A2.centre A3.centre
  measures "d480" distance of A0.centre L27
  measures "d481" distance of A1.centre L27
  measures "d482" distance of A2.centre L27
  measures "d483" distance of A3.centre L27
  measures "d484" distance of A4.centre L27
  measures "d485" distance of A5.centre L27
  measures "d486" distance of A6.centre L27
  measures "d487" distance of A7.centre L27
extrude "Extrude21" cut sketch "Sketch22" against normal through all contours A0 | A1 | A2 | A3 | A4 | A5 | A6 | A7 bodies 1
copy_body "Body->Comp1" bodies 1 removing the originals makes body 11 in component "Baseplate"
copy_body "Body->Comp2" bodies 2 removing the originals makes body 12 in component "Foot corner"
copy_body "Body->Comp3" bodies 3 removing the originals makes body 13 in component "Foot inner"
copy_body "Body->Comp4" bodies 4 removing the originals makes body 14 in component "Motor mount translation"
copy_body "Body->Comp5" bodies 5 removing the originals makes body 15 in component "Bearing mount translation"
copy_body "Body->Comp6" bodies 8 removing the originals makes body 16 in component "Bearing mount egg holder"
copy_body "Body->Comp7" bodies 9 removing the originals makes body 17 in component "Motor mount egg holder"
copy_body "Body->Comp13" bodies 6 removing the originals makes body 18 in component "Mount stopper"
copy_body "Body->Comp14" bodies 10 removing the originals makes body 19 in component "Stabilizer"
copy_body "Body->Comp15" bodies 7 removing the originals makes body 20 in component "Bearing_mount_first"
component "Baseplate" placed x (1, 0, 0) y (0, 1, 0) z (0, 0, 1) at (0, 0, 0)
component "Foot corner" placed x (-1, 0, 0) y (0, 1, 0) z (0, 0, -1) at (435.1655, -14, 127.7164)
component "Foot inner" placed x (0, 0, 1) y (0, 1, 0) z (-1, 0, 0) at (-8.2127, -14, -185.8458)
component "Motor mount translation" placed x (1, 0, 0) y (0, 1, 0) z (0, 0, 1) at (-108.2127, 0, 166.6654)
component "Bearing mount translation" placed x (-1, 0, 0) y (0, 1, 0) z (0, 0, -1) at (159.7073, 0, -319.0915)
component "Bearing mount egg holder" placed x (1, 0, 0) y (0, 1, 0) z (0, 0, 1) at (0, 0, 0)
component "Motor mount egg holder" placed x (1, 0, 0) y (0, 1, 0) z (0, 0, 1) at (-56.2127, 0, -175.8058)
component "Mount stopper" placed x (-1, 0, 0) y (0, 1, 0) z (0, 0, -1) at (163.7073, 0, -389.0915)
component "Stabilizer" placed x (1, 0, 0) y (0, 1, 0) z (0, 0, 1) at (-131.8111, 0, -62.8458)
component "Bearing_mount_first" placed x (1, 0, 0) y (0, 1, 0) z (0, 0, 1) at (-56.2927, 0, 378.3998)
component "Bearing mount egg holder" placed x (1, 0, 0) y (0, 1, 0) z (0, 0, 1) at (0, 0, 0)
component "Motor mount egg holder" placed x (1, 0, 0) y (0, 1, 0) z (0, 0, 1) at (-52.2127, 0, -175.8058)
component "Bearing mount translation" placed x (-1, 0, 0) y (0, 1, 0) z (0, 0, -1) at (155.7073, 0, -319.0915)
component "Bearing mount translation" placed x (1, 0, 0) y (0, 1, 0) z (0, 0, 1) at (-52.2927, 0, 243.3998)
component "Foot corner" placed x (0, 0, -1) y (0, 1, 0) z (1, 0, 0) at (-136.695, -14, 385.6524)
component "Foot corner" placed x (1, 0, 0) y (0, 1, 0) z (0, 0, 1) at (-394.6309, -14, -76.4081)
component "Foot corner" placed x (0, 0, 1) y (0, 1, 0) z (-1, 0, 0) at (177.2295, -14, -334.3441)
component "Stabilizer" placed x (-1, 0, 0) y (0, 1, 0) z (0, 0, -1) at (239.2257, 0, -12.8458)
component "Stabilizer" placed x (1, 0, 0) y (0, 1, 0) z (0, 0, 1) at (-399.7311, 0, -62.8458)
component "Stabilizer" placed x (-1, 0, 0) y (0, 1, 0) z (0, 0, -1) at (239.3057, 0, 114.1542)
equation "thickness = 4 mm"
equation "kerf = 0.08 mm"
equation "distance_axes = 125.5 mm"
equation "d7 = 2 * thickness - kerf"
equation "d8 = 3 * thickness - kerf"
equation "d9 = 2 * thickness - kerf"
equation "d10 = 2 * thickness - kerf"
equation "width_mounts = 50 mm"
equation "d12 = width_mounts - kerf"
equation "d13 = width_mounts - kerf"
equation "d14 = width_mounts - kerf"
equation "d15 = width_mounts - kerf"
equation "d16 = width_mounts - kerf"
equation "d17 = 1 * thickness - kerf"
equation "d18 = d16 / 2"
equation "d19 = d15 / 2"
equation "d20 = d12 / 2"
equation "d21 = d14 / 2"
equation "d22 = d13 / 2"
equation "d23 = d5 - d13 / 2"
equation "d24 = d10"
equation "d26 = d6 - d12 / 2"
equation "d29 = thickness"
equation "height_feet = 10 mm"
equation "d34 = height_feet + thickness + 3 mm"
equation "d42 = -thickness"
equation "d46 = height_feet"
equation "d51 = ( 20 mm - d49 ) / 2"
equation "d58 = 23 mm - kerf"
equation "d59 = d60"
equation "d60 = 4 mm - kerf"
equation "d61 = d60"
equation "d62 = d60"
equation "d64 = d63"
equation "d65 = d63"
equation "d66 = d63"
equation "d67 = d64"
equation "d68 = d66"
equation "d69 = width_mounts - kerf"
equation "d70 = d63 / 2"
equation "d71 = thickness"
equation "d72 = height_translationstage_axis"
equation "d74 = d65 / 2"
equation "d75 = thickness"
equation "d77 = thickness"
equation "d78 = width_mounts - kerf"
equation "bearing_translation_outerdia = 24 mm"
equation "d80 = bearing_translation_outerdia - kerf"
equation "d81 = height_translationstage_axis"
equation "d83 = d78 / 2"
equation "d84 = d78 / 2"
equation "d85 = d78"
equation "d87 = d80 / 2 + 10 mm"
equation "d88 = d78 / 2"
equation "d89 = thickness"
equation "d91 = thickness"
equation "d92 = width_mounts - kerf"
equation "bearing_eggholder_outerdia = 12 mm"
equation "d94 = bearing_eggholder_outerdia - kerf"
equation "d95 = height_eggholder_axis"
equation "height_eggholder_axis = 56 mm"
equation "height_translationstage_axis = 54 mm"
equation "d98 = d92 / 2"
equation "d99 = d92 / 2"
equation "d100 = d94 / 2 + 10 mm"
equation "d101 = d92 / 2"
equation "d102 = thickness"
equation "d104 = thickness"
equation "d105 = 23 mm - kerf"
equation "d106 = 4 mm - kerf"
equation "d108 = d106"
equation "d109 = d106"
equation "d110 = d106"
equation "d111 = d107"
equation "d112 = d111"
equation "d113 = d107"
equation "d114 = d113"
equation "d115 = d111"
equation "d116 = d115 / 2"
equation "d117 = d113 / 2"
equation "d118 = height_eggholder_axis"
equation "d120 = width_mounts - kerf"
equation "d121 = d120 / 2"
equation "d122 = thickness"
equation "d124 = d81 + d77"
equation "d125 = d72 + d71"
equation "d128 = thickness"
equation "d133 = width_mounts"
equation "d138 = screws_dia"
equation "d139 = screws_dia"
equation "d143 = screws_dia"
equation "d144 = screws_dia"
equation "height_screws = 12 mm"
equation "distance_screws = 30 mm"
equation "screws_dia = 3.5 mm"
equation "d149 = height_screws"
equation "d150 = distance_screws"
equation "d151 = d150 / 2"
equation "d152 = d149"
equation "d153 = ( d155 - d154 ) / 2"
equation "d154 = distance_screws"
equation "d156 = height_screws"
equation "d157 = d156"
equation "d160 = height_screws + thickness"
equation "d161 = d160"
equation "d162 = distance_screws"
equation "d163 = screws_dia - kerf"
equation "d164 = screws_dia - kerf"
equation "d165 = ( d166 - d162 ) / 2"
equation "d167 = height_screws + thickness"
equation "d168 = d160"
equation "d169 = distance_screws"
equation "d170 = screws_dia - kerf"
equation "d171 = screws_dia - kerf"